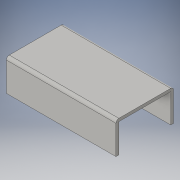
# Autodesk Inventor part: track bracket
Saved by Autodesk Inventor 2016 (Build 200138000, 138)
## iProperties
Created: 2015-10-30
Part Number: track bracket
Material: Generic
Document SubType Name: Modeling
Designer: RoboticsUser
Density: 1 g/cm^3
Appearance: Default
Author: RoboticsUser
Autodesk Inventor part; units mm, degrees
ref_plane "YZ Plane" through (0, 0, 0) normal (1, 0, 0) x (0, 1, 0)
ref_plane "XZ Plane" through (0, 0, 0) normal (0, 1, 0) x (-1, 0, 0)
ref_plane "XY Plane" through (0, 0, 0) normal (0, 0, 1) x (1, 0, 0)
sketch "Sketch1" plane through (0, 0, 0) normal (0, 1, 0) x (-1, 0, 0)
  line L0 (0, 0) -> (-120.65, 0)
  line L1 (-120.65, 0) -> (-120.65, -63.5)
  line L2 (-120.65, -63.5) -> (0, -63.5)
  line L3 (0, -63.5) -> (0, 0)
  dimension "d0" = 120.65
  dimension "d1" = 63.5
  constraints: 8 end point, 2 parallel, 1 horizontal, 1 perpendicular
  measures "d0" distance of L2.end L1.end
  measures "d1" distance of L1.end L0.end
extrude "Extrusion1" add sketch "Sketch1" along normal blind 3.175
sketch "Sketch2" plane through (0, 0, 0) normal (0, 0, 1) x (1, 0, 0)
  line L0 (0, 0) -> (120.65, 0) projected
  line L1 (0, 0) -> (120.65, 0)
  line L2 (120.65, 0) -> (120.65, -31.75)
  line L3 (120.65, -31.75) -> (0, -31.75)
  line L4 (0, -31.75) -> (0, 0)
  dimension "d4" = 31.75
  constraints: 8 end point, 2 parallel, 1 horizontal, 1 perpendicular
  measures "d4" distance of L1.end L2.end
extrude "Extrusion2" add sketch "Sketch2" against normal blind 3.175
sketch "Sketch4" plane through (120.65, 0, -63.5) normal (0, 0, -1) x (-1, 0, 0)
  line L0 (0, -31.75) -> (0, 3.175) projected
  line L1 (120.65, -31.75) -> (120.65, 3.175) projected
  line L2 (0, 3.175) -> (120.65, 3.175)
  line L3 (120.65, 3.175) -> (120.65, -31.75)
  line L4 (120.65, -31.75) -> (0, -31.75)
  line L5 (0, -31.75) -> (0, 3.175)
  point P0 (120.65, 0)
  constraints: 8 end point, 2 parallel, 1 horizontal, 1 perpendicular
extrude "Extrusion4" add sketch "Sketch4" against normal blind 3.175
fillet "Fillet1" radius 3.175 1 edges at (60.325, 3.175, 0)
fillet "Fillet2" radius 3.175 1 edges at (60.325, 3.175, -63.5)
body "Solid1"
